Autodesk Fusion 360 part; units mm, degrees
(part 2 of 2)
sketch "Sketch7" plane through (12.7, 0, 0) normal (1, 0, 0) x (0, 0, -1)
  arc A0 (-250.5905, 407.5484) -> (-267.446, 363.1471) centre (-250.5905, 382.1484) ccw
  line L0 (-250.5905, 407.5484) -> (-117.709, 407.5484)
  arc A1 (-100.8535, 363.147) -> (-117.709, 407.5484) centre (-117.709, 382.1484) ccw
  line L1 (-100.8535, 363.147) -> (-167.2945, 304.2096)
  arc A2 (-201.0055, 304.2097) -> (-167.2945, 304.2096) centre (-184.15, 323.2111) ccw
  line L2 (-201.0055, 304.2097) -> (-267.446, 363.1471)
  arc A3 (-317.5, 185.2722) -> (-289.5997, 168.4029) centre (-298.45, 185.2722) ccw
  line L3 (-317.5, 185.2722) -> (-317.5, 297.278)
  arc A4 (-285.8084, 311.529) -> (-317.5, 297.278) centre (-298.45, 297.278) ccw
  line L4 (-285.8084, 311.529) -> (-229.1614, 261.2792)
  arc A5 (-237.1222, 195.9346) -> (-229.1614, 261.2792) centre (-255.7055, 231.3558) ccw
  line L5 (-237.1222, 195.9346) -> (-289.5997, 168.4029)
  arc A6 (-78.7003, 168.4029) -> (-50.8, 185.2722) centre (-69.85, 185.2722) ccw
  line L6 (-78.7003, 168.4029) -> (-131.1778, 195.9346)
  arc A7 (-139.1386, 261.2792) -> (-131.1778, 195.9346) centre (-112.5945, 231.3558) ccw
  line L7 (-139.1386, 261.2792) -> (-82.4916, 311.529)
  arc A8 (-50.8, 297.278) -> (-82.4916, 311.529) centre (-69.85, 297.278) ccw
  line L8 (-50.8, 297.278) -> (-50.8, 185.2722)
  arc A9 (-128.1151, 96.3984) -> (-119.2648, 132.3177) centre (-128.1151, 115.4484) ccw
  line L9 (-128.1151, 96.3984) -> (-240.1849, 96.3984)
  arc A10 (-249.0352, 132.3177) -> (-240.1849, 96.3984) centre (-240.1849, 115.4484) ccw
  line L10 (-249.0352, 132.3177) -> (-193.0003, 161.7159)
  arc A11 (-175.2997, 161.7159) -> (-193.0003, 161.7159) centre (-184.15, 144.8466) ccw
  line L11 (-175.2997, 161.7159) -> (-119.2648, 132.3177)
  line L12 (0, 426.2984) -> (-368.3, 426.2984)
  line L13 (-368.3, 426.2984) -> (-368.3, 58.2984)
  line L14 (-368.3, 58.2984) -> (0, 58.2984)
  line L15 (0, 58.2984) -> (0, 426.2984)
  arc A12 (-317.5, 530.7784) -> (-298.499, 519.7517) centre (-304.8, 530.7784) ccw
  line L16 (-317.5, 530.7784) -> (-317.5, 573.1917)
  arc A13 (-298.499, 584.2184) -> (-317.5, 573.1917) centre (-304.8, 573.1917) ccw
  line L17 (-298.499, 584.2184) -> (-261.3874, 563.0118)
  arc A14 (-261.3874, 540.9584) -> (-261.3874, 563.0118) centre (-267.6883, 551.9851) ccw
  line L18 (-261.3874, 540.9584) -> (-298.499, 519.7517)
  arc A15 (-177.8417, 530.9452) -> (-190.4433, 530.9455) centre (-184.1427, 519.9185) ccw
  line L19 (-177.8417, 530.9452) -> (-92.3208, 482.075)
  arc A16 (-98.6218, 458.3484) -> (-92.3208, 482.075) centre (-98.6218, 471.0484) ccw
  line L20 (-98.6218, 458.3484) -> (-269.6734, 458.3484)
  arc A17 (-275.974, 482.0754) -> (-269.6734, 458.3484) centre (-269.6734, 471.0484) ccw
  line L21 (-275.974, 482.0754) -> (-190.4433, 530.9455)
  arc A18 (-69.801, 519.7517) -> (-50.8, 530.7784) centre (-63.5, 530.7784) ccw
  line L22 (-69.801, 519.7517) -> (-106.9126, 540.9584)
  arc A19 (-106.9126, 563.0118) -> (-106.9126, 540.9584) centre (-100.6117, 551.9851) ccw
  line L23 (-106.9126, 563.0118) -> (-69.801, 584.2184)
  arc A20 (-50.8, 573.1917) -> (-69.801, 584.2184) centre (-63.5, 573.1917) ccw
  line L24 (-50.8, 573.1917) -> (-50.8, 530.7784)
  arc A21 (-273.321, 661.5484) -> (-279.622, 637.8218) centre (-273.321, 648.8484) ccw
  line L25 (-273.321, 661.5484) -> (-96.4416, 661.5484)
  arc A22 (-90.141, 637.8215) -> (-96.4416, 661.5484) centre (-96.4416, 648.8484) ccw
  line L26 (-90.141, 637.8215) -> (-178.5858, 587.2864)
  arc A23 (-191.1874, 587.2867) -> (-178.5858, 587.2864) centre (-184.8863, 598.3133) ccw
  line L27 (-191.1874, 587.2867) -> (-279.622, 637.8218)
  line L28 (0, 680.2984) -> (-368.3, 680.2984)
  line L29 (-368.3, 680.2984) -> (-368.3, 439.2984)
  line L30 (-368.3, 439.2984) -> (0, 439.2984)
  line L31 (0, 439.2984) -> (0, 680.2984)
  arc A24 (-271.6979, 1150.4984) -> (-276.0278, 1125.8593) centre (-271.6979, 1137.7984) ccw
  line L32 (-271.6979, 1150.4984) -> (-96.602, 1150.4984)
  arc A25 (-92.2722, 1125.8593) -> (-96.602, 1150.4984) centre (-96.602, 1137.7984) ccw
  line L33 (-92.2722, 1125.8593) -> (-179.8202, 1094.1093)
  arc A26 (-188.4798, 1094.1093) -> (-179.8202, 1094.1093) centre (-184.15, 1106.0484) ccw
  line L34 (-188.4798, 1094.1093) -> (-276.0278, 1125.8593)
  line L35 (-368.3, 1074.2984) -> (0, 1074.2984)
  line L36 (0, 1074.2984) -> (0, 1188.2984)
  line L37 (0, 1188.2984) -> (-368.3, 1188.2984)
  line L38 (-368.3, 1188.2984) -> (-368.3, 1074.2984)
  line L39 (0, 1061.2984) -> (-368.3, 1061.2984)
  line L40 (-368.3, 1061.2984) -> (-368.3, 947.2984)
  line L41 (-368.3, 947.2984) -> (0, 947.2984)
  line L42 (0, 947.2984) -> (0, 1061.2984)
  arc A27 (-278.238, 989.935) -> (-271.6979, 966.3484) centre (-271.6979, 979.0484) ccw
  line L43 (-278.238, 989.935) -> (-193.6768, 1040.735)
  arc A28 (-180.8217, 1040.867) -> (-193.6768, 1040.735) centre (-187.1367, 1029.8484) ccw
  line L44 (-180.8217, 1040.867) -> (-92.1848, 990.067)
  arc A29 (-98.4998, 966.3484) -> (-92.1848, 990.067) centre (-98.4998, 979.0484) ccw
  line L45 (-98.4998, 966.3484) -> (-271.6979, 966.3484)
  line L46 (-368.3, 693.2984) -> (0, 693.2984)
  line L47 (0, 693.2984) -> (0, 934.2984)
  line L48 (0, 934.2984) -> (-368.3, 934.2984)
  line L49 (-368.3, 934.2984) -> (-368.3, 693.2984)
  arc A30 (-260.2364, 806.0938) -> (-260.2364, 828.1472) centre (-266.5373, 817.1205) ccw
  line L50 (-260.2364, 806.0938) -> (-297.3478, 784.8873)
  arc A31 (-316.3488, 795.914) -> (-297.3478, 784.8873) centre (-303.6488, 795.914) ccw
  line L51 (-316.3488, 795.914) -> (-316.3488, 838.3271)
  arc A32 (-297.3478, 849.3538) -> (-316.3488, 838.3271) centre (-303.6488, 838.3271) ccw
  line L52 (-297.3478, 849.3538) -> (-260.2364, 828.1472)
  arc A33 (-274.9205, 736.0697) -> (-268.6101, 712.3484) centre (-268.6101, 725.0484) ccw
  line L53 (-274.9205, 736.0697) -> (-189.7746, 784.821)
  arc A34 (-177.1557, 784.8221) -> (-189.7746, 784.821) centre (-183.4642, 773.7997) ccw
  line L54 (-177.1557, 784.8221) -> (-91.977, 736.0708)
  arc A35 (-98.2856, 712.3484) -> (-91.977, 736.0708) centre (-98.2856, 725.0484) ccw
  line L55 (-98.2856, 712.3484) -> (-268.6101, 712.3484)
  arc A36 (-106.7924, 825.1248) -> (-106.7906, 803.0812) centre (-100.482, 814.1035) ccw
  line L56 (-106.7924, 825.1248) -> (-69.8104, 846.2993)
  arc A37 (-50.8, 835.278) -> (-69.8104, 846.2993) centre (-63.5, 835.278) ccw
  line L57 (-50.8, 835.278) -> (-50.8, 792.9372)
  arc A38 (-69.8086, 781.9148) -> (-50.8, 792.9372) centre (-63.5, 792.9372) ccw
  line L58 (-69.8086, 781.9148) -> (-106.7906, 803.0812)
  arc A39 (-272.9377, 915.5484) -> (-279.2463, 891.8261) centre (-272.9377, 902.8484) ccw
  line L59 (-272.9377, 915.5484) -> (-98.8428, 915.5484)
  arc A40 (-92.5324, 891.8271) -> (-98.8428, 915.5484) centre (-98.8428, 902.8484) ccw
  line L60 (-92.5324, 891.8271) -> (-179.5631, 841.9966)
  arc A41 (-192.182, 841.9956) -> (-179.5631, 841.9966) centre (-185.8735, 853.0179) ccw
  line L61 (-192.182, 841.9956) -> (-279.2463, 891.8261)
  line L62 (-368.3, 58.2984) -> (0, 58.2984)
  arc A42 (-271.6979, 1150.4984) -> (-276.0278, 1125.8593) centre (-271.6979, 1137.7984) ccw
  line L63 (-276.0278, 1125.8593) -> (-188.4798, 1094.1093)
  arc A43 (-188.4798, 1094.1093) -> (-179.8202, 1094.1093) centre (-184.15, 1106.0484) ccw
  line L64 (-179.8202, 1094.1093) -> (-92.2722, 1125.8593)
  arc A44 (-92.2722, 1125.8593) -> (-96.602, 1150.4984) centre (-96.602, 1137.7984) ccw
  line L65 (-96.602, 1150.4984) -> (-271.6979, 1150.4984)
  arc A45 (-128.1151, 96.3984) -> (-119.2648, 132.3177) centre (-128.1151, 115.4484) ccw
  line L66 (-119.2648, 132.3177) -> (-175.2997, 161.7159)
  arc A46 (-175.2997, 161.7159) -> (-193.0003, 161.7159) centre (-184.15, 144.8466) ccw
  line L67 (-193.0003, 161.7159) -> (-249.0352, 132.3177)
  arc A47 (-249.0352, 132.3177) -> (-240.1849, 96.3984) centre (-240.1849, 115.4484) ccw
  line L68 (-240.1849, 96.3984) -> (-128.1151, 96.3984)
  arc A48 (-78.7003, 168.4029) -> (-50.8, 185.2722) centre (-69.85, 185.2722) ccw
  line L69 (-50.8, 185.2722) -> (-50.8, 297.278)
  arc A49 (-50.8, 297.278) -> (-82.4916, 311.529) centre (-69.85, 297.278) ccw
  line L70 (-82.4916, 311.529) -> (-139.1386, 261.2792)
  arc A50 (-139.1386, 261.2792) -> (-131.1778, 195.9346) centre (-112.5945, 231.3558) ccw
  line L71 (-131.1778, 195.9346) -> (-78.7003, 168.4029)
  arc A51 (-278.238, 989.935) -> (-271.6979, 966.3484) centre (-271.6979, 979.0484) ccw
  line L72 (-271.6979, 966.3484) -> (-98.4998, 966.3484)
  arc A52 (-98.4998, 966.3484) -> (-92.1848, 990.067) centre (-98.4998, 979.0484) ccw
  line L73 (-92.1848, 990.067) -> (-180.8217, 1040.867)
  arc A53 (-180.8217, 1040.867) -> (-193.6768, 1040.735) centre (-187.1367, 1029.8484) ccw
  line L74 (-193.6768, 1040.735) -> (-278.238, 989.935)
  arc A54 (-317.5, 185.2722) -> (-289.5997, 168.4029) centre (-298.45, 185.2722) ccw
  line L75 (-289.5997, 168.4029) -> (-237.1222, 195.9346)
  arc A55 (-237.1222, 195.9346) -> (-229.1614, 261.2792) centre (-255.7055, 231.3558) ccw
  line L76 (-229.1614, 261.2792) -> (-285.8084, 311.529)
  arc A56 (-285.8084, 311.529) -> (-317.5, 297.278) centre (-298.45, 297.278) ccw
  line L77 (-317.5, 297.278) -> (-317.5, 185.2722)
  arc A57 (-260.2364, 806.0938) -> (-260.2364, 828.1472) centre (-266.5373, 817.1205) ccw
  line L78 (-260.2364, 828.1472) -> (-297.3478, 849.3538)
  arc A58 (-297.3478, 849.3538) -> (-316.3488, 838.3271) centre (-303.6488, 838.3271) ccw
  line L79 (-316.3488, 838.3271) -> (-316.3488, 795.914)
  arc A59 (-316.3488, 795.914) -> (-297.3478, 784.8873) centre (-303.6488, 795.914) ccw
  line L80 (-297.3478, 784.8873) -> (-260.2364, 806.0938)
  arc A60 (-274.9205, 736.0697) -> (-268.6101, 712.3484) centre (-268.6101, 725.0484) ccw
  line L81 (-268.6101, 712.3484) -> (-98.2856, 712.3484)
  arc A61 (-98.2856, 712.3484) -> (-91.977, 736.0708) centre (-98.2856, 725.0484) ccw
  line L82 (-91.977, 736.0708) -> (-177.1557, 784.8221)
  arc A62 (-177.1557, 784.8221) -> (-189.7746, 784.821) centre (-183.4642, 773.7997) ccw
  line L83 (-189.7746, 784.821) -> (-274.9205, 736.0697)
  arc A63 (-106.7924, 825.1248) -> (-106.7906, 803.0812) centre (-100.482, 814.1035) ccw
  line L84 (-106.7906, 803.0812) -> (-69.8086, 781.9148)
  arc A64 (-69.8086, 781.9148) -> (-50.8, 792.9372) centre (-63.5, 792.9372) ccw
  line L85 (-50.8, 792.9372) -> (-50.8, 835.278)
  arc A65 (-50.8, 835.278) -> (-69.8104, 846.2993) centre (-63.5, 835.278) ccw
  line L86 (-69.8104, 846.2993) -> (-106.7924, 825.1248)
  arc A66 (-273.321, 661.5484) -> (-279.622, 637.8218) centre (-273.321, 648.8484) ccw
  line L87 (-279.622, 637.8218) -> (-191.1874, 587.2867)
  arc A67 (-191.1874, 587.2867) -> (-178.5858, 587.2864) centre (-184.8863, 598.3133) ccw
  line L88 (-178.5858, 587.2864) -> (-90.141, 637.8215)
  arc A68 (-90.141, 637.8215) -> (-96.4416, 661.5484) centre (-96.4416, 648.8484) ccw
  line L89 (-96.4416, 661.5484) -> (-273.321, 661.5484)
  arc A69 (-69.801, 519.7517) -> (-50.8, 530.7784) centre (-63.5, 530.7784) ccw
  line L90 (-50.8, 530.7784) -> (-50.8, 573.1917)
  arc A70 (-50.8, 573.1917) -> (-69.801, 584.2184) centre (-63.5, 573.1917) ccw
  line L91 (-69.801, 584.2184) -> (-106.9126, 563.0118)
  arc A71 (-106.9126, 563.0118) -> (-106.9126, 540.9584) centre (-100.6117, 551.9851) ccw
  line L92 (-106.9126, 540.9584) -> (-69.801, 519.7517)
  arc A72 (-177.8417, 530.9452) -> (-190.4433, 530.9455) centre (-184.1427, 519.9185) ccw
  line L93 (-190.4433, 530.9455) -> (-275.974, 482.0754)
  arc A73 (-275.974, 482.0754) -> (-269.6734, 458.3484) centre (-269.6734, 471.0484) ccw
  line L94 (-269.6734, 458.3484) -> (-98.6218, 458.3484)
  arc A74 (-98.6218, 458.3484) -> (-92.3208, 482.075) centre (-98.6218, 471.0484) ccw
  line L95 (-92.3208, 482.075) -> (-177.8417, 530.9452)
  arc A75 (-250.5905, 407.5484) -> (-267.446, 363.1471) centre (-250.5905, 382.1484) ccw
  line L96 (-267.446, 363.1471) -> (-201.0055, 304.2097)
  arc A76 (-201.0055, 304.2097) -> (-167.2945, 304.2096) centre (-184.15, 323.2111) ccw
  line L97 (-167.2945, 304.2096) -> (-100.8535, 363.147)
  arc A77 (-100.8535, 363.147) -> (-117.709, 407.5484) centre (-117.709, 382.1484) ccw
  line L98 (-117.709, 407.5484) -> (-250.5905, 407.5484)
  arc A78 (-317.5, 530.7784) -> (-298.499, 519.7517) centre (-304.8, 530.7784) ccw
  line L99 (-298.499, 519.7517) -> (-261.3874, 540.9584)
  arc A79 (-261.3874, 540.9584) -> (-261.3874, 563.0118) centre (-267.6883, 551.9851) ccw
  line L100 (-261.3874, 563.0118) -> (-298.499, 584.2184)
  arc A80 (-298.499, 584.2184) -> (-317.5, 573.1917) centre (-304.8, 573.1917) ccw
  line L101 (-317.5, 573.1917) -> (-317.5, 530.7784)
  arc A81 (-272.9377, 915.5484) -> (-279.2463, 891.8261) centre (-272.9377, 902.8484) ccw
  line L102 (-279.2463, 891.8261) -> (-192.182, 841.9956)
  arc A82 (-192.182, 841.9956) -> (-179.5631, 841.9966) centre (-185.8735, 853.0179) ccw
  line L103 (-179.5631, 841.9966) -> (-92.5324, 891.8271)
  arc A83 (-92.5324, 891.8271) -> (-98.8428, 915.5484) centre (-98.8428, 902.8484) ccw
  line L104 (-98.8428, 915.5484) -> (-272.9377, 915.5484)
  line L105 (0, 1201.2984) -> (0, 45.5984)
  line L106 (0, 45.5984) -> (-368.3, 45.5984)
  line L107 (-368.3, 45.5984) -> (-368.3, 1201.2984)
  line L108 (-368.3, 1201.2984) -> (0, 1201.2984)
  line L109 (-368.3, 426.2984) -> (0, 426.2984)
  line L110 (0, 426.2984) -> (0, 439.2984)
  line L111 (0, 439.2984) -> (-368.3, 439.2984)
  line L112 (-368.3, 439.2984) -> (-368.3, 426.2984)
extrude "Extrude1" [suppressed]
equation "d151 = ( 7.5 in - 2 in ) / 2"
equation "d168 = ( 7.5 in - 2 in ) / 2"
